Autodesk Fusion 360 part; units mm, degrees
(part 5 of 9)
sketch "草图23" plane through (-116, 0, 0) normal (1, 0, 0) x (0, 1, 0)
  line L0 (-82, 0) -> (-7, 0)
  line L1 (-7, 0) -> (-7, 140)
  line L2 (-7, 140) -> (-82, 140)
  line L3 (-82, 140) -> (-82, 0)
  line L4 (-69.9199, 20.799) -> (-74.25, 18.299)
  line L5 (-74.25, 18.299) -> (-74.25, 13.299)
  line L6 (-74.25, 13.299) -> (-69.9199, 10.799)
  line L7 (-69.9199, 10.799) -> (-65.5897, 13.299)
  line L8 (-65.5897, 13.299) -> (-65.5897, 18.299)
  line L9 (-65.5897, 18.299) -> (-69.9199, 20.799)
  line L10 (-59.7596, 20.799) -> (-64.0897, 18.299)
  line L11 (-64.0897, 18.299) -> (-64.0897, 13.299)
  line L12 (-64.0897, 13.299) -> (-59.7596, 10.799)
  line L13 (-59.7596, 10.799) -> (-55.4295, 13.299)
  line L14 (-55.4295, 13.299) -> (-55.4295, 18.299)
  line L15 (-55.4295, 18.299) -> (-59.7596, 20.799)
  line L16 (-49.5994, 20.799) -> (-53.9295, 18.299)
  line L17 (-53.9295, 18.299) -> (-53.9295, 13.299)
  line L18 (-53.9295, 13.299) -> (-49.5994, 10.799)
  line L19 (-49.5994, 10.799) -> (-45.2692, 13.299)
  line L20 (-45.2692, 13.299) -> (-45.2692, 18.299)
  line L21 (-45.2692, 18.299) -> (-49.5994, 20.799)
  line L22 (-39.4391, 20.799) -> (-43.7692, 18.299)
  line L23 (-43.7692, 18.299) -> (-43.7692, 13.299)
  line L24 (-43.7692, 13.299) -> (-39.4391, 10.799)
  line L25 (-39.4391, 10.799) -> (-35.109, 13.299)
  line L26 (-35.109, 13.299) -> (-35.109, 18.299)
  line L27 (-35.109, 18.299) -> (-39.4391, 20.799)
  line L28 (-29.2789, 20.799) -> (-33.609, 18.299)
  line L29 (-33.609, 18.299) -> (-33.609, 13.299)
  line L30 (-33.609, 13.299) -> (-29.2789, 10.799)
  line L31 (-29.2789, 10.799) -> (-24.9487, 13.299)
  line L32 (-24.9487, 13.299) -> (-24.9487, 18.299)
  line L33 (-24.9487, 18.299) -> (-29.2789, 20.799)
  line L34 (-19.1186, 20.799) -> (-23.4487, 18.299)
  line L35 (-23.4487, 18.299) -> (-23.4487, 13.299)
  line L36 (-23.4487, 13.299) -> (-19.1186, 10.799)
  line L37 (-19.1186, 10.799) -> (-14.7885, 13.299)
  line L38 (-14.7885, 13.299) -> (-14.7885, 18.299)
  line L39 (-14.7885, 18.299) -> (-19.1186, 20.799)
  line L40 (-75, 29.5981) -> (-79.3301, 27.0981)
  line L41 (-79.3301, 27.0981) -> (-79.3301, 22.0981)
  line L42 (-79.3301, 22.0981) -> (-75, 19.5981)
  line L43 (-75, 19.5981) -> (-70.6699, 22.0981)
  line L44 (-70.6699, 22.0981) -> (-70.6699, 27.0981)
  line L45 (-70.6699, 27.0981) -> (-75, 29.5981)
  line L46 (-64.8397, 29.5981) -> (-69.1699, 27.0981)
  line L47 (-69.1699, 27.0981) -> (-69.1699, 22.0981)
  line L48 (-69.1699, 22.0981) -> (-64.8397, 19.5981)
  line L49 (-64.8397, 19.5981) -> (-60.5096, 22.0981)
  line L50 (-60.5096, 22.0981) -> (-60.5096, 27.0981)
  line L51 (-60.5096, 27.0981) -> (-64.8397, 29.5981)
  line L52 (-54.6795, 29.5981) -> (-59.0096, 27.0981)
  line L53 (-59.0096, 27.0981) -> (-59.0096, 22.0981)
  line L54 (-59.0096, 22.0981) -> (-54.6795, 19.5981)
  line L55 (-54.6795, 19.5981) -> (-50.3494, 22.0981)
  line L56 (-50.3494, 22.0981) -> (-50.3494, 27.0981)
  line L57 (-50.3494, 27.0981) -> (-54.6795, 29.5981)
  line L58 (-44.5192, 29.5981) -> (-48.8494, 27.0981)
  line L59 (-48.8494, 27.0981) -> (-48.8494, 22.0981)
  line L60 (-48.8494, 22.0981) -> (-44.5192, 19.5981)
  line L61 (-44.5192, 19.5981) -> (-40.1891, 22.0981)
  line L62 (-40.1891, 22.0981) -> (-40.1891, 27.0981)
  line L63 (-40.1891, 27.0981) -> (-44.5192, 29.5981)
  line L64 (-34.359, 29.5981) -> (-38.6891, 27.0981)
  line L65 (-38.6891, 27.0981) -> (-38.6891, 22.0981)
  line L66 (-38.6891, 22.0981) -> (-34.359, 19.5981)
  line L67 (-34.359, 19.5981) -> (-30.0289, 22.0981)
  line L68 (-30.0289, 22.0981) -> (-30.0289, 27.0981)
  line L69 (-30.0289, 27.0981) -> (-34.359, 29.5981)
  line L70 (-24.1987, 29.5981) -> (-28.5289, 27.0981)
  line L71 (-28.5289, 27.0981) -> (-28.5289, 22.0981)
  line L72 (-28.5289, 22.0981) -> (-24.1987, 19.5981)
  line L73 (-24.1987, 19.5981) -> (-19.8686, 22.0981)
  line L74 (-19.8686, 22.0981) -> (-19.8686, 27.0981)
  line L75 (-19.8686, 27.0981) -> (-24.1987, 29.5981)
  line L76 (-14.0385, 29.5981) -> (-18.3686, 27.0981)
  line L77 (-18.3686, 27.0981) -> (-18.3686, 22.0981)
  line L78 (-18.3686, 22.0981) -> (-14.0385, 19.5981)
  line L79 (-14.0385, 19.5981) -> (-9.7083, 22.0981)
  line L80 (-9.7083, 22.0981) -> (-9.7083, 27.0981)
  line L81 (-9.7083, 27.0981) -> (-14.0385, 29.5981)
  line L82 (-69.9199, 38.3971) -> (-74.25, 35.8971)
  line L83 (-74.25, 35.8971) -> (-74.25, 30.8971)
  line L84 (-74.25, 30.8971) -> (-69.9199, 28.3971)
  line L85 (-69.9199, 28.3971) -> (-65.5897, 30.8971)
  line L86 (-65.5897, 30.8971) -> (-65.5897, 35.8971)
  line L87 (-65.5897, 35.8971) -> (-69.9199, 38.3971)
  line L88 (-59.7596, 38.3971) -> (-64.0897, 35.8971)
  line L89 (-64.0897, 35.8971) -> (-64.0897, 30.8971)
  line L90 (-64.0897, 30.8971) -> (-59.7596, 28.3971)
  line L91 (-59.7596, 28.3971) -> (-55.4295, 30.8971)
  line L92 (-55.4295, 30.8971) -> (-55.4295, 35.8971)
  line L93 (-55.4295, 35.8971) -> (-59.7596, 38.3971)
  line L94 (-49.5994, 38.3971) -> (-53.9295, 35.8971)
  line L95 (-53.9295, 35.8971) -> (-53.9295, 30.8971)
  line L96 (-53.9295, 30.8971) -> (-49.5994, 28.3971)
  line L97 (-49.5994, 28.3971) -> (-45.2692, 30.8971)
  line L98 (-45.2692, 30.8971) -> (-45.2692, 35.8971)
  line L99 (-45.2692, 35.8971) -> (-49.5994, 38.3971)
  line L100 (-39.4391, 38.3971) -> (-43.7692, 35.8971)
  line L101 (-43.7692, 35.8971) -> (-43.7692, 30.8971)
  line L102 (-43.7692, 30.8971) -> (-39.4391, 28.3971)
  line L103 (-39.4391, 28.3971) -> (-35.109, 30.8971)
  line L104 (-35.109, 30.8971) -> (-35.109, 35.8971)
  line L105 (-35.109, 35.8971) -> (-39.4391, 38.3971)
  line L106 (-29.2789, 38.3971) -> (-33.609, 35.8971)
  line L107 (-33.609, 35.8971) -> (-33.609, 30.8971)
  line L108 (-33.609, 30.8971) -> (-29.2789, 28.3971)
  line L109 (-29.2789, 28.3971) -> (-24.9487, 30.8971)
  line L110 (-24.9487, 30.8971) -> (-24.9487, 35.8971)
  line L111 (-24.9487, 35.8971) -> (-29.2789, 38.3971)
  line L112 (-19.1186, 38.3971) -> (-23.4487, 35.8971)
  line L113 (-23.4487, 35.8971) -> (-23.4487, 30.8971)
  line L114 (-23.4487, 30.8971) -> (-19.1186, 28.3971)
  line L115 (-19.1186, 28.3971) -> (-14.7885, 30.8971)
  line L116 (-14.7885, 30.8971) -> (-14.7885, 35.8971)
  line L117 (-14.7885, 35.8971) -> (-19.1186, 38.3971)
  line L118 (-75, 47.1962) -> (-79.3301, 44.6962)
  line L119 (-79.3301, 44.6962) -> (-79.3301, 39.6962)
  line L120 (-79.3301, 39.6962) -> (-75, 37.1962)
  line L121 (-75, 37.1962) -> (-70.6699, 39.6962)
  line L122 (-70.6699, 39.6962) -> (-70.6699, 44.6962)
  line L123 (-70.6699, 44.6962) -> (-75, 47.1962)
  line L124 (-64.8397, 47.1962) -> (-69.1699, 44.6962)
  line L125 (-69.1699, 44.6962) -> (-69.1699, 39.6962)
  line L126 (-69.1699, 39.6962) -> (-64.8397, 37.1962)
  line L127 (-64.8397, 37.1962) -> (-60.5096, 39.6962)
  line L128 (-60.5096, 39.6962) -> (-60.5096, 44.6962)
  line L129 (-60.5096, 44.6962) -> (-64.8397, 47.1962)
  line L130 (-54.6795, 47.1962) -> (-59.0096, 44.6962)
  line L131 (-59.0096, 44.6962) -> (-59.0096, 39.6962)
  line L132 (-59.0096, 39.6962) -> (-54.6795, 37.1962)
  line L133 (-54.6795, 37.1962) -> (-50.3494, 39.6962)
  line L134 (-50.3494, 39.6962) -> (-50.3494, 44.6962)
  line L135 (-50.3494, 44.6962) -> (-54.6795, 47.1962)
  line L136 (-44.5192, 47.1962) -> (-48.8494, 44.6962)
  line L137 (-48.8494, 44.6962) -> (-48.8494, 39.6962)
  line L138 (-48.8494, 39.6962) -> (-44.5192, 37.1962)
  line L139 (-44.5192, 37.1962) -> (-40.1891, 39.6962)
  line L140 (-40.1891, 39.6962) -> (-40.1891, 44.6962)
  line L141 (-40.1891, 44.6962) -> (-44.5192, 47.1962)
  line L142 (-34.359, 47.1962) -> (-38.6891, 44.6962)
  line L143 (-38.6891, 44.6962) -> (-38.6891, 39.6962)
  line L144 (-38.6891, 39.6962) -> (-34.359, 37.1962)
  line L145 (-34.359, 37.1962) -> (-30.0289, 39.6962)
  line L146 (-30.0289, 39.6962) -> (-30.0289, 44.6962)
  line L147 (-30.0289, 44.6962) -> (-34.359, 47.1962)
  line L148 (-24.1987, 47.1962) -> (-28.5289, 44.6962)
  line L149 (-28.5289, 44.6962) -> (-28.5289, 39.6962)
  line L150 (-28.5289, 39.6962) -> (-24.1987, 37.1962)
  line L151 (-24.1987, 37.1962) -> (-19.8686, 39.6962)
  line L152 (-19.8686, 39.6962) -> (-19.8686, 44.6962)
  line L153 (-19.8686, 44.6962) -> (-24.1987, 47.1962)
  line L154 (-14.0385, 47.1962) -> (-18.3686, 44.6962)
  line L155 (-18.3686, 44.6962) -> (-18.3686, 39.6962)
  line L156 (-18.3686, 39.6962) -> (-14.0385, 37.1962)
  line L157 (-14.0385, 37.1962) -> (-9.7083, 39.6962)
  line L158 (-9.7083, 39.6962) -> (-9.7083, 44.6962)
  line L159 (-9.7083, 44.6962) -> (-14.0385, 47.1962)
  line L160 (-69.9199, 55.9952) -> (-74.25, 53.4952)
  line L161 (-74.25, 53.4952) -> (-74.25, 48.4952)
  line L162 (-74.25, 48.4952) -> (-69.9199, 45.9952)
  line L163 (-69.9199, 45.9952) -> (-65.5897, 48.4952)
  line L164 (-65.5897, 48.4952) -> (-65.5897, 53.4952)
  line L165 (-65.5897, 53.4952) -> (-69.9199, 55.9952)
  line L166 (-59.7596, 55.9952) -> (-64.0897, 53.4952)
  line L167 (-64.0897, 53.4952) -> (-64.0897, 48.4952)
  line L168 (-64.0897, 48.4952) -> (-59.7596, 45.9952)
  line L169 (-59.7596, 45.9952) -> (-55.4295, 48.4952)
  line L170 (-55.4295, 48.4952) -> (-55.4295, 53.4952)
  line L171 (-55.4295, 53.4952) -> (-59.7596, 55.9952)
  line L172 (-49.5994, 55.9952) -> (-53.9295, 53.4952)
  line L173 (-53.9295, 53.4952) -> (-53.9295, 48.4952)
  line L174 (-53.9295, 48.4952) -> (-49.5994, 45.9952)
  line L175 (-49.5994, 45.9952) -> (-45.2692, 48.4952)
  line L176 (-45.2692, 48.4952) -> (-45.2692, 53.4952)
  line L177 (-45.2692, 53.4952) -> (-49.5994, 55.9952)
  line L178 (-39.4391, 55.9952) -> (-43.7692, 53.4952)
  line L179 (-43.7692, 53.4952) -> (-43.7692, 48.4952)
  line L180 (-43.7692, 48.4952) -> (-39.4391, 45.9952)
  line L181 (-39.4391, 45.9952) -> (-35.109, 48.4952)
  line L182 (-35.109, 48.4952) -> (-35.109, 53.4952)
  line L183 (-35.109, 53.4952) -> (-39.4391, 55.9952)
  line L184 (-29.2789, 55.9952) -> (-33.609, 53.4952)
  line L185 (-33.609, 53.4952) -> (-33.609, 48.4952)
  line L186 (-33.609, 48.4952) -> (-29.2789, 45.9952)
  line L187 (-29.2789, 45.9952) -> (-24.9487, 48.4952)
  line L188 (-24.9487, 48.4952) -> (-24.9487, 53.4952)
  line L189 (-24.9487, 53.4952) -> (-29.2789, 55.9952)
  line L190 (-19.1186, 55.9952) -> (-23.4487, 53.4952)
  line L191 (-23.4487, 53.4952) -> (-23.4487, 48.4952)
  line L192 (-23.4487, 48.4952) -> (-19.1186, 45.9952)
  line L193 (-19.1186, 45.9952) -> (-14.7885, 48.4952)
  line L194 (-14.7885, 48.4952) -> (-14.7885, 53.4952)
  line L195 (-14.7885, 53.4952) -> (-19.1186, 55.9952)
  line L196 (-75, 64.7942) -> (-79.3301, 62.2942)
  line L197 (-79.3301, 62.2942) -> (-79.3301, 57.2942)
  line L198 (-79.3301, 57.2942) -> (-75, 54.7942)
  line L199 (-75, 54.7942) -> (-70.6699, 57.2942)
  line L200 (-70.6699, 57.2942) -> (-70.6699, 62.2942)
  line L201 (-70.6699, 62.2942) -> (-75, 64.7942)
  line L202 (-64.8397, 64.7942) -> (-69.1699, 62.2942)
  line L203 (-69.1699, 62.2942) -> (-69.1699, 57.2942)
  line L204 (-69.1699, 57.2942) -> (-64.8397, 54.7942)
  line L205 (-64.8397, 54.7942) -> (-60.5096, 57.2942)
  line L206 (-60.5096, 57.2942) -> (-60.5096, 62.2942)
  line L207 (-60.5096, 62.2942) -> (-64.8397, 64.7942)
  line L208 (-54.6795, 64.7942) -> (-59.0096, 62.2942)
  line L209 (-59.0096, 62.2942) -> (-59.0096, 57.2942)
  line L210 (-59.0096, 57.2942) -> (-54.6795, 54.7942)
  line L211 (-54.6795, 54.7942) -> (-50.3494, 57.2942)
  line L212 (-50.3494, 57.2942) -> (-50.3494, 62.2942)
  line L213 (-50.3494, 62.2942) -> (-54.6795, 64.7942)
  line L214 (-44.5192, 64.7942) -> (-48.8494, 62.2942)
  line L215 (-48.8494, 62.2942) -> (-48.8494, 57.2942)
  line L216 (-48.8494, 57.2942) -> (-44.5192, 54.7942)
  line L217 (-44.5192, 54.7942) -> (-40.1891, 57.2942)
  line L218 (-40.1891, 57.2942) -> (-40.1891, 62.2942)
  line L219 (-40.1891, 62.2942) -> (-44.5192, 64.7942)
  line L220 (-34.359, 64.7942) -> (-38.6891, 62.2942)
  line L221 (-38.6891, 62.2942) -> (-38.6891, 57.2942)
  line L222 (-38.6891, 57.2942) -> (-34.359, 54.7942)
  line L223 (-34.359, 54.7942) -> (-30.0289, 57.2942)
  line L224 (-30.0289, 57.2942) -> (-30.0289, 62.2942)
  line L225 (-30.0289, 62.2942) -> (-34.359, 64.7942)
  line L226 (-24.1987, 64.7942) -> (-28.5289, 62.2942)
  line L227 (-28.5289, 62.2942) -> (-28.5289, 57.2942)
  line L228 (-28.5289, 57.2942) -> (-24.1987, 54.7942)
  line L229 (-24.1987, 54.7942) -> (-19.8686, 57.2942)
  line L230 (-19.8686, 57.2942) -> (-19.8686, 62.2942)
  line L231 (-19.8686, 62.2942) -> (-24.1987, 64.7942)
  line L232 (-14.0385, 64.7942) -> (-18.3686, 62.2942)
  line L233 (-18.3686, 62.2942) -> (-18.3686, 57.2942)
  line L234 (-18.3686, 57.2942) -> (-14.0385, 54.7942)
  line L235 (-14.0385, 54.7942) -> (-9.7083, 57.2942)
  line L236 (-9.7083, 57.2942) -> (-9.7083, 62.2942)
  line L237 (-9.7083, 62.2942) -> (-14.0385, 64.7942)
  line L238 (-69.9199, 73.5933) -> (-74.25, 71.0933)
  line L239 (-74.25, 71.0933) -> (-74.25, 66.0933)
  line L240 (-74.25, 66.0933) -> (-69.9199, 63.5933)
  line L241 (-69.9199, 63.5933) -> (-65.5897, 66.0933)
  line L242 (-65.5897, 66.0933) -> (-65.5897, 71.0933)
  line L243 (-65.5897, 71.0933) -> (-69.9199, 73.5933)
  line L244 (-59.7596, 73.5933) -> (-64.0897, 71.0933)
  line L245 (-64.0897, 71.0933) -> (-64.0897, 66.0933)
  line L246 (-64.0897, 66.0933) -> (-59.7596, 63.5933)
  line L247 (-59.7596, 63.5933) -> (-55.4295, 66.0933)
  line L248 (-55.4295, 66.0933) -> (-55.4295, 71.0933)
  line L249 (-55.4295, 71.0933) -> (-59.7596, 73.5933)
  line L250 (-49.5994, 73.5933) -> (-53.9295, 71.0933)
  line L251 (-53.9295, 71.0933) -> (-53.9295, 66.0933)
  line L252 (-53.9295, 66.0933) -> (-49.5994, 63.5933)
  line L253 (-49.5994, 63.5933) -> (-45.2692, 66.0933)
  line L254 (-45.2692, 66.0933) -> (-45.2692, 71.0933)
  line L255 (-45.2692, 71.0933) -> (-49.5994, 73.5933)
  line L256 (-39.4391, 73.5933) -> (-43.7692, 71.0933)
  line L257 (-43.7692, 71.0933) -> (-43.7692, 66.0933)
  line L258 (-43.7692, 66.0933) -> (-39.4391, 63.5933)
  line L259 (-39.4391, 63.5933) -> (-35.109, 66.0933)
  line L260 (-35.109, 66.0933) -> (-35.109, 71.0933)
  line L261 (-35.109, 71.0933) -> (-39.4391, 73.5933)
  line L262 (-29.2789, 73.5933) -> (-33.609, 71.0933)
  line L263 (-33.609, 71.0933) -> (-33.609, 66.0933)
  line L264 (-33.609, 66.0933) -> (-29.2789, 63.5933)
  line L265 (-29.2789, 63.5933) -> (-24.9487, 66.0933)
  line L266 (-24.9487, 66.0933) -> (-24.9487, 71.0933)
  line L267 (-24.9487, 71.0933) -> (-29.2789, 73.5933)
  line L268 (-19.1186, 73.5933) -> (-23.4487, 71.0933)
  line L269 (-23.4487, 71.0933) -> (-23.4487, 66.0933)
  line L270 (-23.4487, 66.0933) -> (-19.1186, 63.5933)
  line L271 (-19.1186, 63.5933) -> (-14.7885, 66.0933)
  line L272 (-14.7885, 66.0933) -> (-14.7885, 71.0933)
  line L273 (-14.7885, 71.0933) -> (-19.1186, 73.5933)
  line L274 (-75, 82.3923) -> (-79.3301, 79.8923)
  line L275 (-79.3301, 79.8923) -> (-79.3301, 74.8923)
  line L276 (-79.3301, 74.8923) -> (-75, 72.3923)
  line L277 (-75, 72.3923) -> (-70.6699, 74.8923)
  line L278 (-70.6699, 74.8923) -> (-70.6699, 79.8923)
  line L279 (-70.6699, 79.8923) -> (-75, 82.3923)
  line L280 (-64.8397, 82.3923) -> (-69.1699, 79.8923)
  line L281 (-69.1699, 79.8923) -> (-69.1699, 74.8923)
  line L282 (-69.1699, 74.8923) -> (-64.8397, 72.3923)
  line L283 (-64.8397, 72.3923) -> (-60.5096, 74.8923)
  line L284 (-60.5096, 74.8923) -> (-60.5096, 79.8923)
  line L285 (-60.5096, 79.8923) -> (-64.8397, 82.3923)
  line L286 (-54.6795, 82.3923) -> (-59.0096, 79.8923)
  line L287 (-59.0096, 79.8923) -> (-59.0096, 74.8923)
  line L288 (-59.0096, 74.8923) -> (-54.6795, 72.3923)
  line L289 (-54.6795, 72.3923) -> (-50.3494, 74.8923)
  line L290 (-50.3494, 74.8923) -> (-50.3494, 79.8923)
  line L291 (-50.3494, 79.8923) -> (-54.6795, 82.3923)
  line L292 (-44.5192, 82.3923) -> (-48.8494, 79.8923)
  line L293 (-48.8494, 79.8923) -> (-48.8494, 74.8923)
  line L294 (-48.8494, 74.8923) -> (-44.5192, 72.3923)
  line L295 (-44.5192, 72.3923) -> (-40.1891, 74.8923)
  line L296 (-40.1891, 74.8923) -> (-40.1891, 79.8923)
  line L297 (-40.1891, 79.8923) -> (-44.5192, 82.3923)
  line L298 (-34.359, 82.3923) -> (-38.6891, 79.8923)
  line L299 (-38.6891, 79.8923) -> (-38.6891, 74.8923)
  line L300 (-38.6891, 74.8923) -> (-34.359, 72.3923)
  line L301 (-34.359, 72.3923) -> (-30.0289, 74.8923)
  line L302 (-30.0289, 74.8923) -> (-30.0289, 79.8923)
  line L303 (-30.0289, 79.8923) -> (-34.359, 82.3923)
  line L304 (-24.1987, 82.3923) -> (-28.5289, 79.8923)
  line L305 (-28.5289, 79.8923) -> (-28.5289, 74.8923)
  line L306 (-28.5289, 74.8923) -> (-24.1987, 72.3923)
  line L307 (-24.1987, 72.3923) -> (-19.8686, 74.8923)
  line L308 (-19.8686, 74.8923) -> (-19.8686, 79.8923)
  line L309 (-19.8686, 79.8923) -> (-24.1987, 82.3923)
  line L310 (-14.0385, 82.3923) -> (-18.3686, 79.8923)
  line L311 (-18.3686, 79.8923) -> (-18.3686, 74.8923)
  line L312 (-18.3686, 74.8923) -> (-14.0385, 72.3923)
  line L313 (-14.0385, 72.3923) -> (-9.7083, 74.8923)
  line L314 (-9.7083, 74.8923) -> (-9.7083, 79.8923)
  line L315 (-9.7083, 79.8923) -> (-14.0385, 82.3923)
  line L316 (-69.9199, 91.1913) -> (-74.25, 88.6913)
  line L317 (-74.25, 88.6913) -> (-74.25, 83.6913)
  line L318 (-74.25, 83.6913) -> (-69.9199, 81.1913)
  line L319 (-69.9199, 81.1913) -> (-65.5897, 83.6913)
  line L320 (-65.5897, 83.6913) -> (-65.5897, 88.6913)
  line L321 (-65.5897, 88.6913) -> (-69.9199, 91.1913)
  line L322 (-59.7596, 91.1913) -> (-64.0897, 88.6913)
  line L323 (-64.0897, 88.6913) -> (-64.0897, 83.6913)
  line L324 (-64.0897, 83.6913) -> (-59.7596, 81.1913)
  line L325 (-59.7596, 81.1913) -> (-55.4295, 83.6913)
  line L326 (-55.4295, 83.6913) -> (-55.4295, 88.6913)
  line L327 (-55.4295, 88.6913) -> (-59.7596, 91.1913)
  line L328 (-49.5994, 91.1913) -> (-53.9295, 88.6913)
  line L329 (-53.9295, 88.6913) -> (-53.9295, 83.6913)
  line L330 (-53.9295, 83.6913) -> (-49.5994, 81.1913)
  line L331 (-49.5994, 81.1913) -> (-45.2692, 83.6913)
  line L332 (-45.2692, 83.6913) -> (-45.2692, 88.6913)
  line L333 (-45.2692, 88.6913) -> (-49.5994, 91.1913)
  line L334 (-39.4391, 91.1913) -> (-43.7692, 88.6913)
  line L335 (-43.7692, 88.6913) -> (-43.7692, 83.6913)
  line L336 (-43.7692, 83.6913) -> (-39.4391, 81.1913)
  line L337 (-39.4391, 81.1913) -> (-35.109, 83.6913)
  line L338 (-35.109, 83.6913) -> (-35.109, 88.6913)
  line L339 (-35.109, 88.6913) -> (-39.4391, 91.1913)
  line L340 (-29.2789, 91.1913) -> (-33.609, 88.6913)
  line L341 (-33.609, 88.6913) -> (-33.609, 83.6913)
  line L342 (-33.609, 83.6913) -> (-29.2789, 81.1913)
  line L343 (-29.2789, 81.1913) -> (-24.9487, 83.6913)
  line L344 (-24.9487, 83.6913) -> (-24.9487, 88.6913)
  line L345 (-24.9487, 88.6913) -> (-29.2789, 91.1913)
  line L346 (-19.1186, 91.1913) -> (-23.4487, 88.6913)
  line L347 (-23.4487, 88.6913) -> (-23.4487, 83.6913)
  line L348 (-23.4487, 83.6913) -> (-19.1186, 81.1913)
  line L349 (-19.1186, 81.1913) -> (-14.7885, 83.6913)
  line L350 (-14.7885, 83.6913) -> (-14.7885, 88.6913)
  line L351 (-14.7885, 88.6913) -> (-19.1186, 91.1913)
  line L352 (-75, 99.9904) -> (-79.3301, 97.4904)
  line L353 (-79.3301, 97.4904) -> (-79.3301, 92.4904)
  line L354 (-79.3301, 92.4904) -> (-75, 89.9904)
  line L355 (-75, 89.9904) -> (-70.6699, 92.4904)
  line L356 (-70.6699, 92.4904) -> (-70.6699, 97.4904)
  line L357 (-70.6699, 97.4904) -> (-75, 99.9904)
  line L358 (-64.8397, 99.9904) -> (-69.1699, 97.4904)
  line L359 (-69.1699, 97.4904) -> (-69.1699, 92.4904)
  line L360 (-69.1699, 92.4904) -> (-64.8397, 89.9904)
  line L361 (-64.8397, 89.9904) -> (-60.5096, 92.4904)
  line L362 (-60.5096, 92.4904) -> (-60.5096, 97.4904)
  line L363 (-60.5096, 97.4904) -> (-64.8397, 99.9904)
  line L364 (-54.6795, 99.9904) -> (-59.0096, 97.4904)
  line L365 (-59.0096, 97.4904) -> (-59.0096, 92.4904)
  line L366 (-59.0096, 92.4904) -> (-54.6795, 89.9904)
  line L367 (-54.6795, 89.9904) -> (-50.3494, 92.4904)
  line L368 (-50.3494, 92.4904) -> (-50.3494, 97.4904)
  line L369 (-50.3494, 97.4904) -> (-54.6795, 99.9904)
  line L370 (-44.5192, 99.9904) -> (-48.8494, 97.4904)
  line L371 (-48.8494, 97.4904) -> (-48.8494, 92.4904)
  line L372 (-48.8494, 92.4904) -> (-44.5192, 89.9904)
  line L373 (-44.5192, 89.9904) -> (-40.1891, 92.4904)
  line L374 (-40.1891, 92.4904) -> (-40.1891, 97.4904)
  line L375 (-40.1891, 97.4904) -> (-44.5192, 99.9904)
  line L376 (-34.359, 99.9904) -> (-38.6891, 97.4904)
  line L377 (-38.6891, 97.4904) -> (-38.6891, 92.4904)
  line L378 (-38.6891, 92.4904) -> (-34.359, 89.9904)
  line L379 (-34.359, 89.9904) -> (-30.0289, 92.4904)
  line L380 (-30.0289, 92.4904) -> (-30.0289, 97.4904)
  line L381 (-30.0289, 97.4904) -> (-34.359, 99.9904)
  line L382 (-24.1987, 99.9904) -> (-28.5289, 97.4904)
  line L383 (-28.5289, 97.4904) -> (-28.5289, 92.4904)
  line L384 (-28.5289, 92.4904) -> (-24.1987, 89.9904)
  line L385 (-24.1987, 89.9904) -> (-19.8686, 92.4904)
  line L386 (-19.8686, 92.4904) -> (-19.8686, 97.4904)
  line L387 (-19.8686, 97.4904) -> (-24.1987, 99.9904)
  line L388 (-14.0385, 99.9904) -> (-18.3686, 97.4904)
  line L389 (-18.3686, 97.4904) -> (-18.3686, 92.4904)
  line L390 (-18.3686, 92.4904) -> (-14.0385, 89.9904)
  line L391 (-14.0385, 89.9904) -> (-9.7083, 92.4904)
  line L392 (-9.7083, 92.4904) -> (-9.7083, 97.4904)
  line L393 (-9.7083, 97.4904) -> (-14.0385, 99.9904)
  line L394 (-69.9199, 108.7894) -> (-74.25, 106.2894)
  line L395 (-74.25, 106.2894) -> (-74.25, 101.2894)
  line L396 (-74.25, 101.2894) -> (-69.9199, 98.7894)
  line L397 (-69.9199, 98.7894) -> (-65.5897, 101.2894)
  line L398 (-65.5897, 101.2894) -> (-65.5897, 106.2894)
  line L399 (-65.5897, 106.2894) -> (-69.9199, 108.7894)
  line L400 (-59.7596, 108.7894) -> (-64.0897, 106.2894)
  line L401 (-64.0897, 106.2894) -> (-64.0897, 101.2894)
  line L402 (-64.0897, 101.2894) -> (-59.7596, 98.7894)
  line L403 (-59.7596, 98.7894) -> (-55.4295, 101.2894)
  line L404 (-55.4295, 101.2894) -> (-55.4295, 106.2894)
  line L405 (-55.4295, 106.2894) -> (-59.7596, 108.7894)
  line L406 (-49.5994, 108.7894) -> (-53.9295, 106.2894)
  line L407 (-53.9295, 106.2894) -> (-53.9295, 101.2894)
  line L408 (-53.9295, 101.2894) -> (-49.5994, 98.7894)
  line L409 (-49.5994, 98.7894) -> (-45.2692, 101.2894)
  line L410 (-45.2692, 101.2894) -> (-45.2692, 106.2894)
  line L411 (-45.2692, 106.2894) -> (-49.5994, 108.7894)
  line L412 (-39.4391, 108.7894) -> (-43.7692, 106.2894)
  line L413 (-43.7692, 106.2894) -> (-43.7692, 101.2894)
  line L414 (-43.7692, 101.2894) -> (-39.4391, 98.7894)
  line L415 (-39.4391, 98.7894) -> (-35.109, 101.2894)
  line L416 (-35.109, 101.2894) -> (-35.109, 106.2894)
  line L417 (-35.109, 106.2894) -> (-39.4391, 108.7894)
  line L418 (-29.2789, 108.7894) -> (-33.609, 106.2894)
  line L419 (-33.609, 106.2894) -> (-33.609, 101.2894)
  line L420 (-33.609, 101.2894) -> (-29.2789, 98.7894)
  line L421 (-29.2789, 98.7894) -> (-24.9487, 101.2894)
  line L422 (-24.9487, 101.2894) -> (-24.9487, 106.2894)
  line L423 (-24.9487, 106.2894) -> (-29.2789, 108.7894)
  line L424 (-19.1186, 108.7894) -> (-23.4487, 106.2894)
  line L425 (-23.4487, 106.2894) -> (-23.4487, 101.2894)
  line L426 (-23.4487, 101.2894) -> (-19.1186, 98.7894)
  line L427 (-19.1186, 98.7894) -> (-14.7885, 101.2894)
  line L428 (-14.7885, 101.2894) -> (-14.7885, 106.2894)
  line L429 (-14.7885, 106.2894) -> (-19.1186, 108.7894)
  line L430 (-75, 117.5885) -> (-79.3301, 115.0885)
  line L431 (-79.3301, 115.0885) -> (-79.3301, 110.0885)
  line L432 (-79.3301, 110.0885) -> (-75, 107.5885)
  line L433 (-75, 107.5885) -> (-70.6699, 110.0885)
  line L434 (-70.6699, 110.0885) -> (-70.6699, 115.0885)
  line L435 (-70.6699, 115.0885) -> (-75, 117.5885)
  line L436 (-64.8397, 117.5885) -> (-69.1699, 115.0885)
  line L437 (-69.1699, 115.0885) -> (-69.1699, 110.0885)
  line L438 (-69.1699, 110.0885) -> (-64.8397, 107.5885)
  line L439 (-64.8397, 107.5885) -> (-60.5096, 110.0885)
  line L440 (-60.5096, 110.0885) -> (-60.5096, 115.0885)
  line L441 (-60.5096, 115.0885) -> (-64.8397, 117.5885)
  line L442 (-54.6795, 117.5885) -> (-59.0096, 115.0885)
  line L443 (-59.0096, 115.0885) -> (-59.0096, 110.0885)
  line L444 (-59.0096, 110.0885) -> (-54.6795, 107.5885)
  line L445 (-54.6795, 107.5885) -> (-50.3494, 110.0885)
  line L446 (-50.3494, 110.0885) -> (-50.3494, 115.0885)
  line L447 (-50.3494, 115.0885) -> (-54.6795, 117.5885)
  line L448 (-44.5192, 117.5885) -> (-48.8494, 115.0885)
  line L449 (-48.8494, 115.0885) -> (-48.8494, 110.0885)
  line L450 (-48.8494, 110.0885) -> (-44.5192, 107.5885)
  line L451 (-44.5192, 107.5885) -> (-40.1891, 110.0885)
  line L452 (-40.1891, 110.0885) -> (-40.1891, 115.0885)
  line L453 (-40.1891, 115.0885) -> (-44.5192, 117.5885)
  line L454 (-34.359, 117.5885) -> (-38.6891, 115.0885)
  line L455 (-38.6891, 115.0885) -> (-38.6891, 110.0885)
  line L456 (-38.6891, 110.0885) -> (-34.359, 107.5885)
  line L457 (-34.359, 107.5885) -> (-30.0289, 110.0885)
  line L458 (-30.0289, 110.0885) -> (-30.0289, 115.0885)
  line L459 (-30.0289, 115.0885) -> (-34.359, 117.5885)
  line L460 (-24.1987, 117.5885) -> (-28.5289, 115.0885)
  line L461 (-28.5289, 115.0885) -> (-28.5289, 110.0885)
  line L462 (-28.5289, 110.0885) -> (-24.1987, 107.5885)
  line L463 (-24.1987, 107.5885) -> (-19.8686, 110.0885)
  line L464 (-19.8686, 110.0885) -> (-19.8686, 115.0885)
  line L465 (-19.8686, 115.0885) -> (-24.1987, 117.5885)
  line L466 (-14.0385, 117.5885) -> (-18.3686, 115.0885)
  line L467 (-18.3686, 115.0885) -> (-18.3686, 110.0885)
  line L468 (-18.3686, 110.0885) -> (-14.0385, 107.5885)
  line L469 (-14.0385, 107.5885) -> (-9.7083, 110.0885)
  line L470 (-9.7083, 110.0885) -> (-9.7083, 115.0885)
  line L471 (-9.7083, 115.0885) -> (-14.0385, 117.5885)
  line L472 (-69.9199, 126.3875) -> (-74.25, 123.8875)
  line L473 (-74.25, 123.8875) -> (-74.25, 118.8875)
  line L474 (-74.25, 118.8875) -> (-69.9199, 116.3875)
  line L475 (-69.9199, 116.3875) -> (-65.5897, 118.8875)
  line L476 (-65.5897, 118.8875) -> (-65.5897, 123.8875)
  line L477 (-65.5897, 123.8875) -> (-69.9199, 126.3875)
  line L478 (-59.7596, 126.3875) -> (-64.0897, 123.8875)
  line L479 (-64.0897, 123.8875) -> (-64.0897, 118.8875)
  line L480 (-64.0897, 118.8875) -> (-59.7596, 116.3875)
  line L481 (-59.7596, 116.3875) -> (-55.4295, 118.8875)
  line L482 (-55.4295, 118.8875) -> (-55.4295, 123.8875)
  line L483 (-55.4295, 123.8875) -> (-59.7596, 126.3875)
  line L484 (-49.5994, 126.3875) -> (-53.9295, 123.8875)
  line L485 (-53.9295, 123.8875) -> (-53.9295, 118.8875)
  line L486 (-53.9295, 118.8875) -> (-49.5994, 116.3875)
  line L487 (-49.5994, 116.3875) -> (-45.2692, 118.8875)
  line L488 (-45.2692, 118.8875) -> (-45.2692, 123.8875)
  line L489 (-45.2692, 123.8875) -> (-49.5994, 126.3875)
  line L490 (-39.4391, 126.3875) -> (-43.7692, 123.8875)
  line L491 (-43.7692, 123.8875) -> (-43.7692, 118.8875)
  line L492 (-43.7692, 118.8875) -> (-39.4391, 116.3875)
  line L493 (-39.4391, 116.3875) -> (-35.109, 118.8875)
  line L494 (-35.109, 118.8875) -> (-35.109, 123.8875)
  line L495 (-35.109, 123.8875) -> (-39.4391, 126.3875)
  line L496 (-29.2789, 126.3875) -> (-33.609, 123.8875)
  line L497 (-33.609, 123.8875) -> (-33.609, 118.8875)
  line L498 (-33.609, 118.8875) -> (-29.2789, 116.3875)
  line L499 (-29.2789, 116.3875) -> (-24.9487, 118.8875)
  line L500 (-24.9487, 118.8875) -> (-24.9487, 123.8875)
  line L501 (-24.9487, 123.8875) -> (-29.2789, 126.3875)
  line L502 (-19.1186, 126.3875) -> (-23.4487, 123.8875)
  line L503 (-23.4487, 123.8875) -> (-23.4487, 118.8875)
  line L504 (-23.4487, 118.8875) -> (-19.1186, 116.3875)
  line L505 (-19.1186, 116.3875) -> (-14.7885, 118.8875)
  line L506 (-14.7885, 118.8875) -> (-14.7885, 123.8875)
  line L507 (-14.7885, 123.8875) -> (-19.1186, 126.3875)
  line L508 (-75, 135.1865) -> (-79.3301, 132.6865)
  line L509 (-79.3301, 132.6865) -> (-79.3301, 127.6865)
  line L510 (-79.3301, 127.6865) -> (-75, 125.1865)
  line L511 (-75, 125.1865) -> (-70.6699, 127.6865)
  line L512 (-70.6699, 127.6865) -> (-70.6699, 132.6865)
  line L513 (-70.6699, 132.6865) -> (-75, 135.1865)
  line L514 (-64.8397, 135.1865) -> (-69.1699, 132.6865)
  line L515 (-69.1699, 132.6865) -> (-69.1699, 127.6865)
  line L516 (-69.1699, 127.6865) -> (-64.8397, 125.1865)
  line L517 (-64.8397, 125.1865) -> (-60.5096, 127.6865)
  line L518 (-60.5096, 127.6865) -> (-60.5096, 132.6865)
  line L519 (-60.5096, 132.6865) -> (-64.8397, 135.1865)
  line L520 (-54.6795, 135.1865) -> (-59.0096, 132.6865)
  line L521 (-59.0096, 132.6865) -> (-59.0096, 127.6865)
  line L522 (-59.0096, 127.6865) -> (-54.6795, 125.1865)
  line L523 (-54.6795, 125.1865) -> (-50.3494, 127.6865)
  line L524 (-50.3494, 127.6865) -> (-50.3494, 132.6865)
  line L525 (-50.3494, 132.6865) -> (-54.6795, 135.1865)
  line L526 (-44.5192, 135.1865) -> (-48.8494, 132.6865)
  line L527 (-48.8494, 132.6865) -> (-48.8494, 127.6865)
  line L528 (-48.8494, 127.6865) -> (-44.5192, 125.1865)
  line L529 (-44.5192, 125.1865) -> (-40.1891, 127.6865)
  line L530 (-40.1891, 127.6865) -> (-40.1891, 132.6865)
  line L531 (-40.1891, 132.6865) -> (-44.5192, 135.1865)
  line L532 (-34.359, 135.1865) -> (-38.6891, 132.6865)
  line L533 (-38.6891, 132.6865) -> (-38.6891, 127.6865)
  line L534 (-38.6891, 127.6865) -> (-34.359, 125.1865)
  line L535 (-34.359, 125.1865) -> (-30.0289, 127.6865)
  line L536 (-30.0289, 127.6865) -> (-30.0289, 132.6865)
  line L537 (-30.0289, 132.6865) -> (-34.359, 135.1865)
  line L538 (-24.1987, 135.1865) -> (-28.5289, 132.6865)
  line L539 (-28.5289, 132.6865) -> (-28.5289, 127.6865)
  line L540 (-28.5289, 127.6865) -> (-24.1987, 125.1865)
  line L541 (-24.1987, 125.1865) -> (-19.8686, 127.6865)
  line L542 (-19.8686, 127.6865) -> (-19.8686, 132.6865)
  line L543 (-19.8686, 132.6865) -> (-24.1987, 135.1865)
  line L544 (-14.0385, 135.1865) -> (-18.3686, 132.6865)
  line L545 (-18.3686, 132.6865) -> (-18.3686, 127.6865)
  line L546 (-18.3686, 127.6865) -> (-14.0385, 125.1865)
  line L547 (-14.0385, 125.1865) -> (-9.7083, 127.6865)
  line L548 (-9.7083, 127.6865) -> (-9.7083, 132.6865)
  line L549 (-9.7083, 132.6865) -> (-14.0385, 135.1865)
extrude "拉伸24" cut sketch "草图23" against normal blind 5 contours L4 L5 L6 L7 L8 L9 | L10 L11 L12 L13 L14 L15 | L16 L17 L18 L19 L20 L21 | L22 L23 L24 L25 L26 L27 | L28 L29 L30 L31 L32 L33 | L34 L35 L36 L37 L38 L39 | L40 L41 L42 L43 L44 L45 | L46 L47 L48 L49 L50 L51 | L52 L53 L54 L55 L56 L57 | L58 L59 L60 L61 L62 L63 | L64 L65 L66 L67 L68 L69 | L70 L71 L72 L73 L74 L75 | L76 L77 L78 L79 L80 L81 | L82 L83 L84 L85 L86 L87 | L88 L89 L90 L91 L92 L93 | L94 L95 L96 L97 L98 L99 | L100 L101 L102 L103 L104 L105 | L106 L107 L108 L109 L110 L111 | L112 L113 L114 L115 L116 L117 | L118 L119 L120 L121 L122 L123 | L124 L125 L126 L127 L128 L129 | L130 L131 L132 L133 L134 L135 | L136 L137 L138 L139 L140 L141 | L142 L143 L144 L145 L146 L147 | L148 L149 L150 L151 L152 L153 | L154 L155 L156 L157 L158 L159 | L160 L161 L162 L163 L164 L165 | L166 L167 L168 L169 L170 L171 | L172 L173 L174 L175 L176 L177 | L178 L179 L180 L181 L182 L183 | L184 L185 L186 L187 L188 L189 | L190 L191 L192 L193 L194 L195 | L196 L197 L198 L199 L200 L201 | L202 L203 L204 L205 L206 L207 | L208 L209 L210 L211 L212 L213 | L214 L215 L216 L217 L218 L219 | L220 L221 L222 L223 L224 L225 | L226 L227 L228 L229 L230 L231 | L232 L233 L234 L235 L236 L237 | L238 L239 L240 L241 L242 L243 | L244 L245 L246 L247 L248 L249 | L250 L251 L252 L253 L254 L255 | L256 L257 L258 L259 L260 L261 | L262 L263 L264 L265 L266 L267 | L268 L269 L270 L271 L272 L273 | L274 L275 L276 L277 L278 L279 | L280 L281 L282 L283 L284 L285 | L286 L287 L288 L289 L290 L291 | L292 L293 L294 L295 L296 L297 | L298 L299 L300 L301 L302 L303 | L304 L305 L306 L307 L308 L309 | L310 L311 L312 L313 L314 L315 | L316 L317 L318 L319 L320 L321 | L322 L323 L324 L325 L326 L327 | L328 L329 L330 L331 L332 L333 | L334 L335 L336 L337 L338 L339 | L340 L341 L342 L343 L344 L345 | L346 L347 L348 L349 L350 L351 | L352 L353 L354 L355 L356 L357 | L358 L359 L360 L361 L362 L363 | L364 L365 L366 L367 L368 L369 | L370 L371 L372 L373 L374 L375 | L376 L377 L378 L379 L380 L381 | L382 L383 L384 L385 L386 L387 | L388 L389 L390 L391 L392 L393 | L394 L395 L396 L397 L398 L399 | L400 L401 L402 L403 L404 L405 | L406 L407 L408 L409 L410 L411 | L412 L413 L414 L415 L416 L417 | L418 L419 L420 L421 L422 L423 | L424 L425 L426 L427 L428 L429 | L430 L431 L432 L433 L434 L435 | L436 L437 L438 L439 L440 L441 | L442 L443 L444 L445 L446 L447 | L448 L449 L450 L451 L452 L453 | L454 L455 L456 L457 L458 L459 | L460 L461 L462 L463 L464 L465 | L466 L467 L468 L469 L470 L471 | L472 L473 L474 L475 L476 L477 | L478 L479 L480 L481 L482 L483 | L484 L485 L486 L487 L488 L489 | L490 L491 L492 L493 L494 L495 | L496 L497 L498 L499 L500 L501 | L502 L503 L504 L505 L506 L507 | L508 L509 L510 L511 L512 L513 | L514 L515 L516 L517 L518 L519 | L520 L521 L522 L523 L524 L525 | L526 L527 L528 L529 L530 L531 | L532 L533 L534 L535 L536 L537 | L538 L539 L540 L541 L542 L543 | L544 L545 L546 L547 L548 L549 bodies 1 3
sketch "草图24" plane through (-116, 0, 0) normal (1, 0, 0) x (0, 1, 0)
  line L0 (-38.6891, 132.6865) -> (-34.359, 135.1865)
  line L1 (-34.359, 135.1865) -> (-30.0289, 132.6865)
  line L2 (-30.0289, 132.6865) -> (-30.0289, 127.6865)
  line L3 (-30.0289, 127.6865) -> (-34.359, 125.1865)
  line L4 (-34.359, 125.1865) -> (-38.6891, 127.6865)
  line L5 (-38.6891, 127.6865) -> (-38.6891, 132.6865)
  line L6 (-79.3301, 132.6865) -> (-75, 135.1865)
  line L7 (-75, 135.1865) -> (-70.6699, 132.6865)
  line L8 (-70.6699, 132.6865) -> (-70.6699, 127.6865)
  line L9 (-70.6699, 127.6865) -> (-75, 125.1865)
  line L10 (-75, 125.1865) -> (-79.3301, 127.6865)
  line L11 (-79.3301, 127.6865) -> (-79.3301, 132.6865)
  line L12 (-53.9295, 123.8875) -> (-49.5994, 126.3875)
  line L13 (-49.5994, 126.3875) -> (-45.2692, 123.8875)
  line L14 (-45.2692, 123.8875) -> (-45.2692, 118.8875)
  line L15 (-45.2692, 118.8875) -> (-49.5994, 116.3875)
  line L16 (-49.5994, 116.3875) -> (-53.9295, 118.8875)
  line L17 (-53.9295, 118.8875) -> (-53.9295, 123.8875)
  line L18 (-28.5289, 115.0885) -> (-24.1987, 117.5885)
  line L19 (-24.1987, 117.5885) -> (-19.8686, 115.0885)
  line L20 (-19.8686, 115.0885) -> (-19.8686, 110.0885)
  line L21 (-19.8686, 110.0885) -> (-24.1987, 107.5885)
  line L22 (-24.1987, 107.5885) -> (-28.5289, 110.0885)
  line L23 (-28.5289, 110.0885) -> (-28.5289, 115.0885)
  line L24 (-69.1699, 115.0885) -> (-64.8397, 117.5885)
  line L25 (-64.8397, 117.5885) -> (-60.5096, 115.0885)
  line L26 (-60.5096, 115.0885) -> (-60.5096, 110.0885)
  line L27 (-60.5096, 110.0885) -> (-64.8397, 107.5885)
  line L28 (-64.8397, 107.5885) -> (-69.1699, 110.0885)
  line L29 (-69.1699, 110.0885) -> (-69.1699, 115.0885)
  line L30 (-43.7692, 106.2894) -> (-39.4391, 108.7894)
  line L31 (-39.4391, 108.7894) -> (-35.109, 106.2894)
  line L32 (-35.109, 106.2894) -> (-35.109, 101.2894)
  line L33 (-35.109, 101.2894) -> (-39.4391, 98.7894)
  line L34 (-39.4391, 98.7894) -> (-43.7692, 101.2894)
  line L35 (-43.7692, 101.2894) -> (-43.7692, 106.2894)
  line L36 (-18.3686, 97.4904) -> (-14.0385, 99.9904)
  line L37 (-14.0385, 99.9904) -> (-9.7083, 97.4904)
  line L38 (-9.7083, 97.4904) -> (-9.7083, 92.4904)
  line L39 (-9.7083, 92.4904) -> (-14.0385, 89.9904)
  line L40 (-14.0385, 89.9904) -> (-18.3686, 92.4904)
  line L41 (-18.3686, 92.4904) -> (-18.3686, 97.4904)
  line L42 (-59.0096, 97.4904) -> (-54.6795, 99.9904)
  line L43 (-54.6795, 99.9904) -> (-50.3494, 97.4904)
  line L44 (-50.3494, 97.4904) -> (-50.3494, 92.4904)
  line L45 (-50.3494, 92.4904) -> (-54.6795, 89.9904)
  line L46 (-54.6795, 89.9904) -> (-59.0096, 92.4904)
  line L47 (-59.0096, 92.4904) -> (-59.0096, 97.4904)
  line L48 (-33.609, 88.6913) -> (-29.2789, 91.1913)
  line L49 (-29.2789, 91.1913) -> (-24.9487, 88.6913)
  line L50 (-24.9487, 88.6913) -> (-24.9487, 83.6913)
  line L51 (-24.9487, 83.6913) -> (-29.2789, 81.1913)
  line L52 (-29.2789, 81.1913) -> (-33.609, 83.6913)
  line L53 (-33.609, 83.6913) -> (-33.609, 88.6913)
  line L54 (-74.25, 88.6913) -> (-69.9199, 91.1913)
  line L55 (-69.9199, 91.1913) -> (-65.5897, 88.6913)
  line L56 (-65.5897, 88.6913) -> (-65.5897, 83.6913)
  line L57 (-65.5897, 83.6913) -> (-69.9199, 81.1913)
  line L58 (-69.9199, 81.1913) -> (-74.25, 83.6913)
  line L59 (-74.25, 83.6913) -> (-74.25, 88.6913)
  line L60 (-48.8494, 79.8923) -> (-44.5192, 82.3923)
  line L61 (-44.5192, 82.3923) -> (-40.1891, 79.8923)
  line L62 (-40.1891, 79.8923) -> (-40.1891, 74.8923)
  line L63 (-40.1891, 74.8923) -> (-44.5192, 72.3923)
  line L64 (-44.5192, 72.3923) -> (-48.8494, 74.8923)
  line L65 (-48.8494, 74.8923) -> (-48.8494, 79.8923)
  line L66 (-23.4487, 71.0933) -> (-19.1186, 73.5933)
  line L67 (-19.1186, 73.5933) -> (-14.7885, 71.0933)
  line L68 (-14.7885, 71.0933) -> (-14.7885, 66.0933)
  line L69 (-14.7885, 66.0933) -> (-19.1186, 63.5933)
  line L70 (-19.1186, 63.5933) -> (-23.4487, 66.0933)
  line L71 (-23.4487, 66.0933) -> (-23.4487, 71.0933)
  line L72 (-64.0897, 71.0933) -> (-59.7596, 73.5933)
  line L73 (-59.7596, 73.5933) -> (-55.4295, 71.0933)
  line L74 (-55.4295, 71.0933) -> (-55.4295, 66.0933)
  line L75 (-55.4295, 66.0933) -> (-59.7596, 63.5933)
  line L76 (-59.7596, 63.5933) -> (-64.0897, 66.0933)
  line L77 (-64.0897, 66.0933) -> (-64.0897, 71.0933)
  line L78 (-38.6891, 62.2942) -> (-34.359, 64.7942)
  line L79 (-34.359, 64.7942) -> (-30.0289, 62.2942)
  line L80 (-30.0289, 62.2942) -> (-30.0289, 57.2942)
  line L81 (-30.0289, 57.2942) -> (-34.359, 54.7942)
  line L82 (-34.359, 54.7942) -> (-38.6891, 57.2942)
  line L83 (-38.6891, 57.2942) -> (-38.6891, 62.2942)
  line L84 (-79.3301, 62.2942) -> (-75, 64.7942)
  line L85 (-75, 64.7942) -> (-70.6699, 62.2942)
  line L86 (-70.6699, 62.2942) -> (-70.6699, 57.2942)
  line L87 (-70.6699, 57.2942) -> (-75, 54.7942)
  line L88 (-75, 54.7942) -> (-79.3301, 57.2942)
  line L89 (-79.3301, 57.2942) -> (-79.3301, 62.2942)
  line L90 (-53.9295, 53.4952) -> (-49.5994, 55.9952)
  line L91 (-49.5994, 55.9952) -> (-45.2692, 53.4952)
  line L92 (-45.2692, 53.4952) -> (-45.2692, 48.4952)
  line L93 (-45.2692, 48.4952) -> (-49.5994, 45.9952)
  line L94 (-49.5994, 45.9952) -> (-53.9295, 48.4952)
  line L95 (-53.9295, 48.4952) -> (-53.9295, 53.4952)
  line L96 (-28.5289, 44.6962) -> (-24.1987, 47.1962)
  line L97 (-24.1987, 47.1962) -> (-19.8686, 44.6962)
  line L98 (-19.8686, 44.6962) -> (-19.8686, 39.6962)
  line L99 (-19.8686, 39.6962) -> (-24.1987, 37.1962)
  line L100 (-24.1987, 37.1962) -> (-28.5289, 39.6962)
  line L101 (-28.5289, 39.6962) -> (-28.5289, 44.6962)
  line L102 (-69.1699, 44.6962) -> (-64.8397, 47.1962)
  line L103 (-64.8397, 47.1962) -> (-60.5096, 44.6962)
  line L104 (-60.5096, 44.6962) -> (-60.5096, 39.6962)
  line L105 (-60.5096, 39.6962) -> (-64.8397, 37.1962)
  line L106 (-64.8397, 37.1962) -> (-69.1699, 39.6962)
  line L107 (-69.1699, 39.6962) -> (-69.1699, 44.6962)
  line L108 (-43.7692, 35.8971) -> (-39.4391, 38.3971)
  line L109 (-39.4391, 38.3971) -> (-35.109, 35.8971)
  line L110 (-35.109, 35.8971) -> (-35.109, 30.8971)
  line L111 (-35.109, 30.8971) -> (-39.4391, 28.3971)
  line L112 (-39.4391, 28.3971) -> (-43.7692, 30.8971)
  line L113 (-43.7692, 30.8971) -> (-43.7692, 35.8971)
  line L114 (-18.3686, 27.0981) -> (-14.0385, 29.5981)
  line L115 (-14.0385, 29.5981) -> (-9.7083, 27.0981)
  line L116 (-9.7083, 27.0981) -> (-9.7083, 22.0981)
  line L117 (-9.7083, 22.0981) -> (-14.0385, 19.5981)
  line L118 (-14.0385, 19.5981) -> (-18.3686, 22.0981)
  line L119 (-18.3686, 22.0981) -> (-18.3686, 27.0981)
  line L120 (-59.0096, 27.0981) -> (-54.6795, 29.5981)
  line L121 (-54.6795, 29.5981) -> (-50.3494, 27.0981)
  line L122 (-50.3494, 27.0981) -> (-50.3494, 22.0981)
  line L123 (-50.3494, 22.0981) -> (-54.6795, 19.5981)
  line L124 (-54.6795, 19.5981) -> (-59.0096, 22.0981)
  line L125 (-59.0096, 22.0981) -> (-59.0096, 27.0981)
  line L126 (-33.609, 18.299) -> (-29.2789, 20.799)
  line L127 (-29.2789, 20.799) -> (-24.9487, 18.299)
  line L128 (-24.9487, 18.299) -> (-24.9487, 13.299)
  line L129 (-24.9487, 13.299) -> (-29.2789, 10.799)
  line L130 (-29.2789, 10.799) -> (-33.609, 13.299)
  line L131 (-33.609, 13.299) -> (-33.609, 18.299)
  line L132 (-74.25, 18.299) -> (-69.9199, 20.799)
  line L133 (-69.9199, 20.799) -> (-65.5897, 18.299)
  line L134 (-65.5897, 18.299) -> (-65.5897, 13.299)
  line L135 (-65.5897, 13.299) -> (-69.9199, 10.799)
  line L136 (-69.9199, 10.799) -> (-74.25, 13.299)
  line L137 (-74.25, 13.299) -> (-74.25, 18.299)
  line L138 (-43.7692, 18.299) -> (-39.4391, 20.799)
  line L139 (-39.4391, 20.799) -> (-35.109, 18.299)
  line L140 (-35.109, 18.299) -> (-35.109, 13.299)
  line L141 (-35.109, 13.299) -> (-39.4391, 10.799)
  line L142 (-39.4391, 10.799) -> (-43.7692, 13.299)
  line L143 (-43.7692, 13.299) -> (-43.7692, 18.299)
  line L144 (-69.1699, 27.0981) -> (-64.8397, 29.5981)
  line L145 (-64.8397, 29.5981) -> (-60.5096, 27.0981)
  line L146 (-60.5096, 27.0981) -> (-60.5096, 22.0981)
  line L147 (-60.5096, 22.0981) -> (-64.8397, 19.5981)
  line L148 (-64.8397, 19.5981) -> (-69.1699, 22.0981)
  line L149 (-69.1699, 22.0981) -> (-69.1699, 27.0981)
  line L150 (-28.5289, 27.0981) -> (-24.1987, 29.5981)
  line L151 (-24.1987, 29.5981) -> (-19.8686, 27.0981)
  line L152 (-19.8686, 27.0981) -> (-19.8686, 22.0981)
  line L153 (-19.8686, 22.0981) -> (-24.1987, 19.5981)
  line L154 (-24.1987, 19.5981) -> (-28.5289, 22.0981)
  line L155 (-28.5289, 22.0981) -> (-28.5289, 27.0981)
  line L156 (-53.9295, 35.8971) -> (-49.5994, 38.3971)
  line L157 (-49.5994, 38.3971) -> (-45.2692, 35.8971)
  line L158 (-45.2692, 35.8971) -> (-45.2692, 30.8971)
  line L159 (-45.2692, 30.8971) -> (-49.5994, 28.3971)
  line L160 (-49.5994, 28.3971) -> (-53.9295, 30.8971)
  line L161 (-53.9295, 30.8971) -> (-53.9295, 35.8971)
  line L162 (-79.3301, 44.6962) -> (-75, 47.1962)
  line L163 (-75, 47.1962) -> (-70.6699, 44.6962)
  line L164 (-70.6699, 44.6962) -> (-70.6699, 39.6962)
  line L165 (-70.6699, 39.6962) -> (-75, 37.1962)
  line L166 (-75, 37.1962) -> (-79.3301, 39.6962)
  line L167 (-79.3301, 39.6962) -> (-79.3301, 44.6962)
  line L168 (-38.6891, 44.6962) -> (-34.359, 47.1962)
  line L169 (-34.359, 47.1962) -> (-30.0289, 44.6962)
  line L170 (-30.0289, 44.6962) -> (-30.0289, 39.6962)
  line L171 (-30.0289, 39.6962) -> (-34.359, 37.1962)
  line L172 (-34.359, 37.1962) -> (-38.6891, 39.6962)
  line L173 (-38.6891, 39.6962) -> (-38.6891, 44.6962)
  line L174 (-64.0897, 53.4952) -> (-59.7596, 55.9952)
  line L175 (-59.7596, 55.9952) -> (-55.4295, 53.4952)
  line L176 (-55.4295, 53.4952) -> (-55.4295, 48.4952)
  line L177 (-55.4295, 48.4952) -> (-59.7596, 45.9952)
  line L178 (-59.7596, 45.9952) -> (-64.0897, 48.4952)
  line L179 (-64.0897, 48.4952) -> (-64.0897, 53.4952)
  line L180 (-23.4487, 53.4952) -> (-19.1186, 55.9952)
  line L181 (-19.1186, 55.9952) -> (-14.7885, 53.4952)
  line L182 (-14.7885, 53.4952) -> (-14.7885, 48.4952)
  line L183 (-14.7885, 48.4952) -> (-19.1186, 45.9952)
  line L184 (-19.1186, 45.9952) -> (-23.4487, 48.4952)
  line L185 (-23.4487, 48.4952) -> (-23.4487, 53.4952)
  line L186 (-48.8494, 62.2942) -> (-44.5192, 64.7942)
  line L187 (-44.5192, 64.7942) -> (-40.1891, 62.2942)
  line L188 (-40.1891, 62.2942) -> (-40.1891, 57.2942)
  line L189 (-40.1891, 57.2942) -> (-44.5192, 54.7942)
  line L190 (-44.5192, 54.7942) -> (-48.8494, 57.2942)
  line L191 (-48.8494, 57.2942) -> (-48.8494, 62.2942)
  line L192 (-74.25, 71.0933) -> (-69.9199, 73.5933)
  line L193 (-69.9199, 73.5933) -> (-65.5897, 71.0933)
  line L194 (-65.5897, 71.0933) -> (-65.5897, 66.0933)
  line L195 (-65.5897, 66.0933) -> (-69.9199, 63.5933)
  line L196 (-69.9199, 63.5933) -> (-74.25, 66.0933)
  line L197 (-74.25, 66.0933) -> (-74.25, 71.0933)
  line L198 (-33.609, 71.0933) -> (-29.2789, 73.5933)
  line L199 (-29.2789, 73.5933) -> (-24.9487, 71.0933)
  line L200 (-24.9487, 71.0933) -> (-24.9487, 66.0933)
  line L201 (-24.9487, 66.0933) -> (-29.2789, 63.5933)
  line L202 (-29.2789, 63.5933) -> (-33.609, 66.0933)
  line L203 (-33.609, 66.0933) -> (-33.609, 71.0933)
  line L204 (-59.0096, 79.8923) -> (-54.6795, 82.3923)
  line L205 (-54.6795, 82.3923) -> (-50.3494, 79.8923)
  line L206 (-50.3494, 79.8923) -> (-50.3494, 74.8923)
  line L207 (-50.3494, 74.8923) -> (-54.6795, 72.3923)
  line L208 (-54.6795, 72.3923) -> (-59.0096, 74.8923)
  line L209 (-59.0096, 74.8923) -> (-59.0096, 79.8923)
  line L210 (-18.3686, 79.8923) -> (-14.0385, 82.3923)
  line L211 (-14.0385, 82.3923) -> (-9.7083, 79.8923)
  line L212 (-9.7083, 79.8923) -> (-9.7083, 74.8923)
  line L213 (-9.7083, 74.8923) -> (-14.0385, 72.3923)
  line L214 (-14.0385, 72.3923) -> (-18.3686, 74.8923)
  line L215 (-18.3686, 74.8923) -> (-18.3686, 79.8923)
  line L216 (-43.7692, 88.6913) -> (-39.4391, 91.1913)
  line L217 (-39.4391, 91.1913) -> (-35.109, 88.6913)
  line L218 (-35.109, 88.6913) -> (-35.109, 83.6913)
  line L219 (-35.109, 83.6913) -> (-39.4391, 81.1913)
  line L220 (-39.4391, 81.1913) -> (-43.7692, 83.6913)
  line L221 (-43.7692, 83.6913) -> (-43.7692, 88.6913)
  line L222 (-69.1699, 97.4904) -> (-64.8397, 99.9904)
  line L223 (-64.8397, 99.9904) -> (-60.5096, 97.4904)
  line L224 (-60.5096, 97.4904) -> (-60.5096, 92.4904)
  line L225 (-60.5096, 92.4904) -> (-64.8397, 89.9904)
  line L226 (-64.8397, 89.9904) -> (-69.1699, 92.4904)
  line L227 (-69.1699, 92.4904) -> (-69.1699, 97.4904)
  line L228 (-28.5289, 97.4904) -> (-24.1987, 99.9904)
  line L229 (-24.1987, 99.9904) -> (-19.8686, 97.4904)
  line L230 (-19.8686, 97.4904) -> (-19.8686, 92.4904)
  line L231 (-19.8686, 92.4904) -> (-24.1987, 89.9904)
  line L232 (-24.1987, 89.9904) -> (-28.5289, 92.4904)
  line L233 (-28.5289, 92.4904) -> (-28.5289, 97.4904)
  line L234 (-53.9295, 106.2894) -> (-49.5994, 108.7894)
  line L235 (-49.5994, 108.7894) -> (-45.2692, 106.2894)
  line L236 (-45.2692, 106.2894) -> (-45.2692, 101.2894)
  line L237 (-45.2692, 101.2894) -> (-49.5994, 98.7894)
  line L238 (-49.5994, 98.7894) -> (-53.9295, 101.2894)
  line L239 (-53.9295, 101.2894) -> (-53.9295, 106.2894)
  line L240 (-79.3301, 115.0885) -> (-75, 117.5885)
  line L241 (-75, 117.5885) -> (-70.6699, 115.0885)
  line L242 (-70.6699, 115.0885) -> (-70.6699, 110.0885)
  line L243 (-70.6699, 110.0885) -> (-75, 107.5885)
  line L244 (-75, 107.5885) -> (-79.3301, 110.0885)
  line L245 (-79.3301, 110.0885) -> (-79.3301, 115.0885)
  line L246 (-38.6891, 115.0885) -> (-34.359, 117.5885)
  line L247 (-34.359, 117.5885) -> (-30.0289, 115.0885)
  line L248 (-30.0289, 115.0885) -> (-30.0289, 110.0885)
  line L249 (-30.0289, 110.0885) -> (-34.359, 107.5885)
  line L250 (-34.359, 107.5885) -> (-38.6891, 110.0885)
  line L251 (-38.6891, 110.0885) -> (-38.6891, 115.0885)
  line L252 (-64.0897, 123.8875) -> (-59.7596, 126.3875)
  line L253 (-59.7596, 126.3875) -> (-55.4295, 123.8875)
  line L254 (-55.4295, 123.8875) -> (-55.4295, 118.8875)
  line L255 (-55.4295, 118.8875) -> (-59.7596, 116.3875)
  line L256 (-59.7596, 116.3875) -> (-64.0897, 118.8875)
  line L257 (-64.0897, 118.8875) -> (-64.0897, 123.8875)
  line L258 (-23.4487, 123.8875) -> (-19.1186, 126.3875)
  line L259 (-19.1186, 126.3875) -> (-14.7885, 123.8875)
  line L260 (-14.7885, 123.8875) -> (-14.7885, 118.8875)
  line L261 (-14.7885, 118.8875) -> (-19.1186, 116.3875)
  line L262 (-19.1186, 116.3875) -> (-23.4487, 118.8875)
  line L263 (-23.4487, 118.8875) -> (-23.4487, 123.8875)
  line L264 (-48.8494, 132.6865) -> (-44.5192, 135.1865)
  line L265 (-44.5192, 135.1865) -> (-40.1891, 132.6865)
  line L266 (-40.1891, 132.6865) -> (-40.1891, 127.6865)
  line L267 (-40.1891, 127.6865) -> (-44.5192, 125.1865)
  line L268 (-44.5192, 125.1865) -> (-48.8494, 127.6865)
  line L269 (-48.8494, 127.6865) -> (-48.8494, 132.6865)
  line L270 (-28.5289, 132.6865) -> (-24.1987, 135.1865)
  line L271 (-24.1987, 135.1865) -> (-19.8686, 132.6865)
  line L272 (-19.8686, 132.6865) -> (-19.8686, 127.6865)
  line L273 (-19.8686, 127.6865) -> (-24.1987, 125.1865)
  line L274 (-24.1987, 125.1865) -> (-28.5289, 127.6865)
  line L275 (-28.5289, 127.6865) -> (-28.5289, 132.6865)
  line L276 (-69.1699, 132.6865) -> (-64.8397, 135.1865)
  line L277 (-64.8397, 135.1865) -> (-60.5096, 132.6865)
  line L278 (-60.5096, 132.6865) -> (-60.5096, 127.6865)
  line L279 (-60.5096, 127.6865) -> (-64.8397, 125.1865)
  line L280 (-64.8397, 125.1865) -> (-69.1699, 127.6865)
  line L281 (-69.1699, 127.6865) -> (-69.1699, 132.6865)
  line L282 (-43.7692, 123.8875) -> (-39.4391, 126.3875)
  line L283 (-39.4391, 126.3875) -> (-35.109, 123.8875)
  line L284 (-35.109, 123.8875) -> (-35.109, 118.8875)
  line L285 (-35.109, 118.8875) -> (-39.4391, 116.3875)
  line L286 (-39.4391, 116.3875) -> (-43.7692, 118.8875)
  line L287 (-43.7692, 118.8875) -> (-43.7692, 123.8875)
  line L288 (-18.3686, 115.0885) -> (-14.0385, 117.5885)
  line L289 (-14.0385, 117.5885) -> (-9.7083, 115.0885)
  line L290 (-9.7083, 115.0885) -> (-9.7083, 110.0885)
  line L291 (-9.7083, 110.0885) -> (-14.0385, 107.5885)
  line L292 (-14.0385, 107.5885) -> (-18.3686, 110.0885)
  line L293 (-18.3686, 110.0885) -> (-18.3686, 115.0885)
  line L294 (-59.0096, 115.0885) -> (-54.6795, 117.5885)
  line L295 (-54.6795, 117.5885) -> (-50.3494, 115.0885)
  line L296 (-50.3494, 115.0885) -> (-50.3494, 110.0885)
  line L297 (-50.3494, 110.0885) -> (-54.6795, 107.5885)
  line L298 (-54.6795, 107.5885) -> (-59.0096, 110.0885)
  line L299 (-59.0096, 110.0885) -> (-59.0096, 115.0885)
  line L300 (-33.609, 106.2894) -> (-29.2789, 108.7894)
  line L301 (-29.2789, 108.7894) -> (-24.9487, 106.2894)
  line L302 (-24.9487, 106.2894) -> (-24.9487, 101.2894)
  line L303 (-24.9487, 101.2894) -> (-29.2789, 98.7894)
  line L304 (-29.2789, 98.7894) -> (-33.609, 101.2894)
  line L305 (-33.609, 101.2894) -> (-33.609, 106.2894)
  line L306 (-74.25, 106.2894) -> (-69.9199, 108.7894)
  line L307 (-69.9199, 108.7894) -> (-65.5897, 106.2894)
  line L308 (-65.5897, 106.2894) -> (-65.5897, 101.2894)